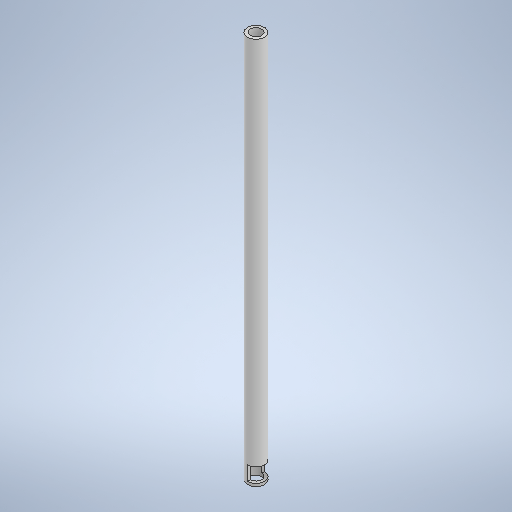
# Autodesk Inventor part: rurkadoczujnika
Saved by Autodesk Inventor 2025 (Build 290162000, 162)
## iProperties
Created: 2025-01-01
Part Number: rurkadoczujnika
Material: Ogólny
Document SubType Name: Modeling
Designer: Laptop
Density: 1 g/cm^3
Appearance: Domyślna
Author: Laptop
Autodesk Inventor part; units mm, degrees
ref_plane "YZ Plane" through (0, 0, 0) normal (1, 0, 0) x (0, 1, 0)
ref_plane "XZ Plane" through (0, 0, 0) normal (0, 1, 0) x (-1, 0, 0)
ref_plane "XY Plane" through (0, 0, 0) normal (0, 0, 1) x (1, 0, 0)
sketch "Szkic1" plane through (0, 0, 0) normal (0, 1, 0) x (-1, 0, 0)
  circle A0 centre (0, 0) radius 3
  circle A1 centre (0, 0) radius 2
  dimension "d0" = 6
  dimension "d1" = 4
  constraints: 2 centre point, 2 coincident
  measures "d0" diameter of A0
  measures "d1" diameter of A1
extrude "Wyciągnięcie proste1" add sketch "Szkic1" along normal blind 135
sketch "Szkic2" plane through (0, 0, 0) normal (0, -1, 0) x (1, 0, 0)
  circle A0 centre (0, 0) radius 2 projected
  circle A1 centre (0, 0) radius 3
  dimension "d4" = 6
  constraints: 1 centre point, 1 coincident
  measures "d4" diameter of A1
sketch "Szkic3" plane through (0, 0, 0) normal (0, -1, 0) x (1, 0, 0)
  circle A0 centre (0, 0) radius 3 projected
  line L0 (-0.7678, 2.9001) -> (-0.7678, 1.8467)
  circle A1 centre (0, 0) radius 2 projected
  line L1 (-0.7678, -1.8467) -> (-0.7678, -2.9012)
  line L2 (0.7678, 2.9001) -> (0.7678, 1.8467)
  line L3 (0.7678, -1.8467) -> (0.7678, -2.9001)
  line L4 (-5.8889, 4.1288) -> (-0.7678, 4.1288)
  line L5 (-0.7678, 4.1288) -> (-0.7678, -5.0287)
  line L6 (-0.7678, -5.0287) -> (-5.8889, -5.0287)
  line L7 (-5.8889, -5.0287) -> (-5.8889, 4.1288)
  line L8 (0.0074, 4.1288) -> (6.1006, 4.1288)
  line L9 (6.1006, 4.1288) -> (6.1006, -5.0287)
  line L10 (6.1006, -5.0287) -> (0.0074, -5.0287)
  line L11 (0.0074, -5.0287) -> (0.0074, 4.1288)
  point P0 (-0.7678, -2.9001)
  constraints: 24 end point, 7 point on circle, 6 point on line, 4 parallel, 2 horizontal, 2 perpendicular, 2 vertical
extrude "Wyciągnięcie proste2" cut sketch "Szkic3" against normal blind 5 contours A0 L3 A1 L2 | A0 L11 L8 L9 L10 | L2 A1 L11 A0 | A0 L11 A1 L3 | A1 L11 | A0 L5 L6 L7 L4
extrude "Wyciągnięcie proste3" add sketch "Szkic2" along normal blind 1 contours A0 | A1
sketch "Szkic4" plane through (0, -1, 0) normal (0, -1, 0) x (1, 0, 0)
  circle A0 centre (0, 0) radius 2
  dimension "d9" = 4
  constraints: 1 centre point, 1 coincident
  measures "d9" diameter of A0
extrude "Wyciągnięcie proste4" cut sketch "Szkic4" against normal blind 5
